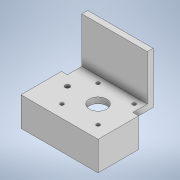
# Autodesk Inventor part: Base Motor X1
Saved by Autodesk Inventor 2021 (Build 250183000, 183)
## iProperties
Created: 2023-01-26
Part Number: Base Motor X1
Material: Genérico
Document SubType Name: Modeling
Designer: Diego.labarca
Density: 1 g/cm^3
Appearance: Valor por defecto
Author: Diego.labarca
Autodesk Inventor part; units mm, degrees
ref_plane "YZ Plane" through (0, 0, 0) normal (1, 0, 0) x (0, 1, 0)
ref_plane "XZ Plane" through (0, 0, 0) normal (0, 1, 0) x (-1, 0, 0)
sketch "Boceto1" plane through (0, 0, 0) normal (0, 1, 0) x (-1, 0, 0)
  line L0 (21.15, 21.15) -> (-21.15, 21.15)
  line L1 (-21.15, 21.15) -> (-21.15, -21.15)
  line L2 (-21.15, -21.15) -> (21.15, -21.15)
  line L3 (21.15, -21.15) -> (21.15, 21.15)
  line L4 (0, 0) -> (3.2885, 0)
  line L5 (0, 0) -> (0, -4.7563)
  circle A0 centre (0, 0) radius 7.5
  line L6 (21.15, -21.15) -> (35, -21.15)
  line L7 (35, -21.15) -> (35, 21.15)
  line L8 (35, 21.15) -> (21.15, 21.15)
  line L9 (21.15, 21.15) -> (21.15, -21.15)
  dimension "d0" = 42.3
  dimension "d1" = 42.3
  dimension "d26" = 15
  dimension "d35" = 35
  constraints: 20 end point, 4 parallel, 3 horizontal, 2 perpendicular, 1 centre point, 1 coincident, 1 vertical, 2 other
  measures "d0" distance of L2.end L1.end
  measures "d1" distance of L1.end L0.end
  measures "d26" diameter of A0
  measures "d35" distance from line of L4.start L7
extrude "Extrusión1" add sketch "Boceto1" along normal blind 5
sketch "Boceto2" plane through (0, 5, 0) normal (0, 1, 0) x (1, 0, 0)
  circle A0 centre (-15.5, 15.5) radius 1.5
  point P0 (0, 0)
  dimension "d4" = 3
  dimension "d5" = 15.5
  dimension "d6" = 15.5
  constraints: 1 centre point
  measures "d4" diameter of A0
  measures "d5" horizontal distance of point (0, 0) A0.centre
  measures "d6" horizontal distance of point (0, 0) A0.centre
extrude "Extrusión2" cut sketch "Boceto2" against normal through all
pattern_circular "Patrón circular1" count 4 over 360 about axis through (0, -10, 0) along (0, 1, 0) of "Extrusión2"
sketch "Boceto7" plane through (0, 0, 0) normal (0, -1, 0) x (1, 0, 0)
  circle A0 centre (-26.3, 0) radius 2
  point P0 (0, 0)
  dimension "d31" = 4
  dimension "d32" = 26.3
  constraints: 1 centre point
  measures "d31" diameter of A0
  measures "d32" distance of point (0, 0) A0.centre
extrude "Extrusión7" cut sketch "Boceto7" against normal through all
sketch "Boceto8" plane through (21.15, 0, -21.15) normal (0, 0, -1) x (-1, 0, 0)
  line L0 (0, 0) -> (0, 5) projected
  line L1 (0, 0) -> (56.15, 0)
  line L2 (56.15, 0) -> (56.15, 44)
  line L3 (56.15, 44) -> (0, 44)
  line L4 (0, 44) -> (0, 0)
  line L5 (0, 5) -> (56.15, 5) projected
  point P0 (21.15, 0)
  dimension "d36" = 39
  constraints: 8 end point, 2 parallel, 1 horizontal, 1 perpendicular
  measures "d36" distance between parallel lines of L3 L5
extrude "Extrusión8" add sketch "Boceto8" along normal blind 5
ref_plane "Plano de trabajo1" through (0, -15, 0) normal (0, -1, 0) x (1, 0, 0)
sketch "Boceto9" plane through (0, -15, 0) normal (0, -1, 0) x (1, 0, 0)
  line L0 (21.15, 21.15) -> (21.15, -26.15) projected
  line L1 (-35, 21.15) -> (21.15, 21.15) projected
  line L2 (-35, 21.15) -> (-35, -26.15) projected
  circle A0 centre (0, 0) radius 2.5
  circle A1 centre (-26.3, 0) radius 2
  line L3 (-35, -21.15) -> (-35, 21.15) projected
  line L4 (21.15, -26.15) -> (-35, -26.15)
  line L5 (-35, -26.15) -> (-35, -8.65)
  line L6 (-35, -8.65) -> (21.15, -8.65)
  line L7 (21.15, -8.65) -> (21.15, -26.15)
  point P0 (-35, -26.15)
  point P1 (21.15, -8.65)
  dimension "d45" = 5
  dimension "d46" = 17.5
  constraints: 8 end point, 2 centre point, 2 parallel, 1 coincident, 1 horizontal, 1 perpendicular, 1 point on line
  measures "d45" diameter of A0
  measures "d46" distance of L4.end L5.end
extrude "Extrusión9" add sketch "Boceto9" along normal blind 5 contours L0 L6 L2 L1
sketch "Boceto10" plane through (0, -20, 0) normal (0, -1, 0) x (1, 0, 0)
  line L0 (-35, -8.65) -> (21.15, -8.65) projected
  line L1 (21.15, -8.65) -> (26.15, -8.65)
  line L2 (26.15, -8.65) -> (26.15, 26.15)
  line L3 (26.15, 26.15) -> (-40, 26.15)
  line L4 (-40, 26.15) -> (-40, -8.65)
  line L5 (-40, -8.65) -> (-35, -8.65)
  line L6 (-35, -21.15) -> (-35, 21.15) projected
  line L7 (21.15, 21.15) -> (-35, 21.15) projected
  line L8 (21.15, -8.65) -> (21.15, 21.15) projected
  line L9 (-35, 21.15) -> (-35, -8.65) projected
  point P0 (0, 0)
  dimension "d47" = 5
  dimension "d48" = 5
  dimension "d49" = 5
  constraints: 10 end point, 3 perpendicular, 3 point on line, 1 horizontal
  measures "d47" distance of L0.end L1.end
  measures "d48" distance between parallel lines of L3 L7
  measures "d49" distance between parallel lines of L6 L4
extrude "Extrusión10" add sketch "Boceto10" against normal up to surface (25 mm away) contours L5 L4 L3 L2 L1 L8 L7 L6
equation "\"d0\" = d1"
equation "\"d6\" = d5"
equation "\"d48\" = d47"
equation "\"d49\" = d47"
